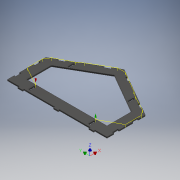
# Autodesk Inventor part: BA15
Saved by Autodesk Inventor 2017 (Build 210142000, 142)
## iProperties
Created: 2019-05-29
Part Number: BA15
Material: Wood (Cherry)
Document SubType Name: Modeling
Designer: Dell
Density: 0.63 g/cm^3
Appearance: Smooth - Black
Mass: 254.003 g
Surface Area: 1468.73 cm^2
Volume: 403.179 cm^3
Author: Dell
Autodesk Inventor part; units mm, degrees
ref_plane "YZ Plane" through (0, 0, 0) normal (1, 0, 0) x (0, 1, 0)
ref_plane "XZ Plane" through (0, 0, 0) normal (0, 1, 0) x (-1, 0, 0)
ref_plane "XY Plane" through (0, 0, 0) normal (0, 0, 1) x (1, 0, 0)
sketch "Sketch1" plane through (0, 0, 0) normal (0, 0, 1) x (1, 0, 0)
  line L0 (0, 0) -> (0, 201.9592)
  line L1 (0, 201.9592) -> (262.89, 353.7388)
  line L2 (262.89, 353.7388) -> (525.78, 201.9592)
  line L3 (525.78, 201.9592) -> (525.78, 0)
  line L4 (525.78, 0) -> (0, 0)
  point P0 (262.89, 0)
  dimension "d0" = 525.78
  dimension "d1" = 120
  dimension "d2" = 201.9592
  constraints: 10 end point, 1 horizontal alignment, 1 midpoint, 1 parallel, 1 perpendicular, 1 vertical, 1 vertical alignment
  measures "d0" distance of L3.end L0.start
  measures "d1" angle of L2 L1
  measures "d2" distance of L0.start L0.end
extrude "Extrusion1" add sketch "Sketch1" along normal blind 6.35
sketch "Sketch3" plane through (0, 0, 6.35) normal (0, 0, 1) x (1, 0, 0)
  line L0 (50.8, 180.4886) -> (474.98, 180.4886)
  line L1 (474.98, 180.4886) -> (474.98, 50.8)
  line L2 (474.98, 50.8) -> (50.8, 50.8)
  line L3 (50.8, 50.8) -> (50.8, 180.4886)
  line L4 (0, 201.9592) -> (0, 0) projected
  line L5 (50.8, 180.4886) -> (262.89, 302.9388)
  line L6 (262.89, 302.9388) -> (474.98, 180.4886)
  line L7 (525.78, 0) -> (0, 0) projected
  point P0 (262.89, 353.7388)
  point P1 (262.89, 180.4886)
  dimension "d15" = 120
  dimension "d16" = 50.8
  dimension "d17" = 50.8
  dimension "d18" = 50.8
  constraints: 12 end point, 2 parallel, 2 vertical alignment, 1 horizontal, 1 midpoint, 1 perpendicular
  measures "d15" angle of L6 L5
  measures "d16" distance between parallel lines of L4 L3
  measures "d17" distance between parallel lines of L7 L2
  measures "d18" distance of point (262.89, 353.739) L5.end
extrude "Extrusion3" cut sketch "Sketch3" against normal through all
sketch "Sketch4" plane through (0, 0, 6.35) normal (0, 0, 1) x (1, 0, 0)
  line L0 (525.78, 163.8592) -> (518.16, 163.8592)
  line L1 (518.16, 163.8592) -> (518.16, 138.4592)
  line L2 (518.16, 138.4592) -> (525.78, 138.4592)
  line L3 (525.78, 138.4592) -> (525.78, 163.8592)
  line L4 (525.78, 201.9592) -> (525.78, 0) projected
  line L5 (525.78, 36.8592) -> (518.16, 36.8592)
  line L6 (518.16, 36.8592) -> (518.16, 62.2592)
  line L7 (518.16, 62.2592) -> (525.78, 62.2592)
  line L8 (525.78, 62.2592) -> (525.78, 36.8592)
  line L9 (518.16, 151.1592) -> (518.16, 49.5592) construction
  line L10 (262.89, 353.7388) -> (262.89, 385.1225)
  line L11 (0, 163.8592) -> (7.62, 163.8592)
  line L12 (7.62, 163.8592) -> (7.62, 138.4592)
  line L13 (7.62, 138.4592) -> (0, 138.4592)
  line L14 (0, 138.4592) -> (0, 163.8592)
  line L15 (0, 201.9592) -> (0, 0)
  line L16 (0, 36.8592) -> (7.62, 36.8592)
  line L17 (7.62, 36.8592) -> (7.62, 62.2592)
  line L18 (7.62, 62.2592) -> (0, 62.2592)
  line L19 (0, 62.2592) -> (0, 36.8592)
  line L20 (7.62, 151.1592) -> (7.62, 49.5592) construction
  point P0 (0, 0)
  dimension "d19" = 38.1
  dimension "d20" = 25.4
  dimension "d21" = 25.4
  dimension "d22" = 7.62
  dimension "d23" = 101.6
  constraints: 40 end point, 12 symmetric about line, 4 parallel, 4 point on line, 2 horizontal, 2 midpoint, 2 perpendicular, 1 vertical, 1 vertical alignment
  measures "d19" vertical distance of L4.start L0.end
  measures "d20" distance of L0.end L1.end
  measures "d21" distance of L5.end L6.end
  measures "d22" distance of L0.start L0.end
  measures "d23" distance of L9.start L9.end
extrude "Extrusion4" cut sketch "Sketch4" against normal through all
sketch "Sketch5" plane through (0, 0, 6.35) normal (0, 0, 1) x (1, 0, 0)
  line L0 (302.5368, 322.0499) -> (306.3468, 328.649)
  line L1 (306.3468, 328.649) -> (328.3439, 315.949)
  line L2 (328.3439, 315.949) -> (324.5339, 309.3499)
  line L3 (324.5339, 309.3499) -> (302.5368, 322.0499)
  line L4 (460.3261, 239.749) -> (456.5161, 233.1499)
  line L5 (456.5161, 233.1499) -> (478.5132, 220.4499)
  line L6 (478.5132, 220.4499) -> (482.3232, 227.049)
  line L7 (482.3232, 227.049) -> (460.3261, 239.749)
  line L8 (525.78, 201.9592) -> (262.89, 353.7388) construction
  line L9 (313.5353, 315.6999) -> (467.5147, 226.7999) construction
  line L10 (390.525, 271.2499) -> (394.335, 277.849) construction
  line L11 (262.89, 353.7388) -> (525.78, 201.9592) construction
  line L12 (262.89, 353.7388) -> (262.89, 420.8284)
  line L13 (223.2432, 322.0499) -> (219.4332, 328.649)
  line L14 (219.4332, 328.649) -> (197.4361, 315.949)
  line L15 (197.4361, 315.949) -> (201.2461, 309.3499)
  line L16 (201.2461, 309.3499) -> (223.2432, 322.0499)
  line L17 (65.4539, 239.749) -> (69.2639, 233.1499)
  line L18 (69.2639, 233.1499) -> (47.2668, 220.4499)
  line L19 (47.2668, 220.4499) -> (43.4568, 227.049)
  line L20 (43.4568, 227.049) -> (65.4539, 239.749)
  line L21 (212.2447, 315.6999) -> (58.2653, 226.7999) construction
  line L22 (135.255, 271.2499) -> (131.445, 277.849) construction
  point P0 (0, 0)
  point P1 (0, 201.9592)
  dimension "d26" = 7.62
  dimension "d27" = 25.4
  dimension "d28" = 25.4
  dimension "d30" = 152.4
  constraints: 42 end point, 13 symmetric about line, 5 midpoint, 5 parallel, 4 perpendicular, 3 point on line, 1 vertical
  measures "d26" distance of L0.start L0.end
  measures "d27" distance of L2.end L0.start
  measures "d28" distance of L4.end L5.end
  measures "d30" distance of L4.end L2.end
extrude "Extrusion5" cut sketch "Sketch5" against normal through all
sketch "Sketch6" plane through (0, 0, 6.35) normal (0, 0, 1) x (1, 0, 0)
  line L0 (525.78, 0) -> (0, 0) projected
  line L1 (250.19, 0) -> (275.59, 0)
  line L2 (275.59, 0) -> (275.59, -7.62)
  line L3 (275.59, -7.62) -> (250.19, -7.62)
  line L4 (250.19, -7.62) -> (250.19, 0)
  line L5 (62.69, 0) -> (88.09, 0)
  line L6 (88.09, 0) -> (88.09, -7.62)
  line L7 (88.09, -7.62) -> (62.69, -7.62)
  line L8 (62.69, -7.62) -> (62.69, 0)
  line L9 (437.69, 0) -> (463.09, 0)
  line L10 (463.09, 0) -> (463.09, -7.62)
  line L11 (463.09, -7.62) -> (437.69, -7.62)
  line L12 (437.69, -7.62) -> (437.69, 0)
  line L13 (75.39, -7.62) -> (450.39, -7.62) construction
  point P0 (262.89, 0)
  point P1 (262.89, -7.62)
  dimension "d33" = 25.4
  dimension "d34" = 7.62
  dimension "d35" = 25.4
  dimension "d36" = 25.4
  dimension "d37" = 375
  constraints: 26 end point, 6 midpoint, 6 parallel, 3 horizontal, 3 perpendicular, 3 point on line, 2 horizontal alignment
  measures "d33" distance of L2.end L3.end
  measures "d34" distance of L1.end L2.end
  measures "d35" distance of L6.end L7.end
  measures "d36" distance of L10.end L11.end
  measures "d37" distance of L13.start L13.end
extrude "Extrusion6" add sketch "Sketch6" against normal blind 6.35
sketch "Sketch7" plane through (0, 0, 6.35) normal (0, 0, 1) x (1, 0, 0)
  line L0 (101.6, 245.2342) -> (107.95, 245.2342)
  line L1 (107.95, 245.2342) -> (107.95, 219.8342)
  line L2 (107.95, 219.8342) -> (101.6, 219.8342)
  line L3 (101.6, 219.8342) -> (101.6, 245.2342)
  line L4 (107.95, 38.1) -> (101.6, 38.1)
  line L5 (101.6, 38.1) -> (101.6, 12.7)
  line L6 (101.6, 12.7) -> (107.95, 12.7)
  line L7 (107.95, 12.7) -> (107.95, 38.1)
  line L8 (0, 0) -> (62.69, 0) projected
  line L9 (0, 36.8592) -> (0, 0) projected
  line L10 (262.89, 353.7388) -> (262.89, 392.9766)
  line L11 (424.18, 245.2342) -> (417.83, 245.2342)
  line L12 (417.83, 245.2342) -> (417.83, 219.8342)
  line L13 (417.83, 219.8342) -> (424.18, 219.8342)
  line L14 (424.18, 219.8342) -> (424.18, 245.2342)
  line L15 (417.83, 38.1) -> (424.18, 38.1)
  line L16 (424.18, 38.1) -> (424.18, 12.7)
  line L17 (424.18, 12.7) -> (417.83, 12.7)
  line L18 (417.83, 12.7) -> (417.83, 38.1)
  point P0 (104.775, 219.8342)
  point P1 (104.775, 38.1)
  point P2 (421.005, 219.8342)
  point P3 (421.005, 38.1)
  point P4 (463.09, 0)
  dimension "d40" = 6.35
  dimension "d41" = 25.4
  dimension "d42" = 12.7
  dimension "d43" = 25.4
  dimension "d44" = 101.6
  dimension "d45" = 181.7342
  constraints: 34 end point, 11 symmetric about line, 4 parallel, 4 point on line, 2 horizontal, 2 midpoint, 2 perpendicular, 2 vertical alignment, 1 vertical
  measures "d40" distance of L1.end L2.end
  measures "d41" distance of L0.end L1.end
  measures "d42" distance from line of L8 L5.end
  measures "d43" distance of L6.end L4.start
  measures "d44" distance between parallel lines of L9 L5
  measures "d45" distance of point (104.775, 38.1) point (104.775, 219.834)
extrude "Extrusion7" cut sketch "Sketch7" against normal through all
sketch "Sketch8" plane through (0, 0, 6.35) normal (0, 0, 1) x (1, 0, 0)
  circle A0 centre (3.175, 100.3592) radius 2.25
  line L0 (417.83, 219.8342) -> (417.83, 245.2342) construction
  line L1 (417.83, 245.2342) -> (424.18, 245.2342) construction
  line L2 (424.18, 245.2342) -> (424.18, 219.8342) construction
  line L3 (424.18, 219.8342) -> (417.83, 219.8342) construction
  line L4 (101.6, 219.8342) -> (101.6, 245.2342) construction
  line L5 (101.6, 245.2342) -> (107.95, 245.2342) construction
  line L6 (107.95, 245.2342) -> (107.95, 219.8342) construction
  line L7 (107.95, 219.8342) -> (101.6, 219.8342) construction
  line L8 (101.6, 12.7) -> (101.6, 38.1) construction
  line L9 (101.6, 38.1) -> (107.95, 38.1) construction
  line L10 (107.95, 38.1) -> (107.95, 12.7) construction
  line L11 (107.95, 12.7) -> (101.6, 12.7) construction
  line L12 (417.83, 12.7) -> (417.83, 38.1) construction
  line L13 (417.83, 38.1) -> (424.18, 38.1) construction
  line L14 (424.18, 38.1) -> (424.18, 12.7) construction
  line L15 (424.18, 12.7) -> (417.83, 12.7) construction
  line L16 (50.8, 50.8) -> (50.8, 180.4886) construction
  line L17 (50.8, 180.4886) -> (262.89, 302.9388) construction
  line L18 (262.89, 302.9388) -> (474.98, 180.4886) construction
  line L19 (474.98, 180.4886) -> (474.98, 50.8) construction
  line L20 (474.98, 50.8) -> (50.8, 50.8) construction
  line L21 (219.4332, 328.649) -> (223.2432, 322.0499) construction
  line L22 (223.2432, 322.0499) -> (201.2461, 309.3499) construction
  line L23 (201.2461, 309.3499) -> (197.4361, 315.949) construction
  line L24 (197.4361, 315.949) -> (65.4539, 239.749) construction
  line L25 (65.4539, 239.749) -> (69.2639, 233.1499) construction
  line L26 (69.2639, 233.1499) -> (47.2668, 220.4499) construction
  line L27 (47.2668, 220.4499) -> (43.4568, 227.049) construction
  line L28 (43.4568, 227.049) -> (0, 201.9592) construction
  line L29 (0, 201.9592) -> (0, 163.8592) construction
  line L30 (0, 163.8592) -> (7.62, 163.8592) construction
  line L31 (7.62, 163.8592) -> (7.62, 138.4592) construction
  line L32 (7.62, 138.4592) -> (0, 138.4592) construction
  line L33 (0, 138.4592) -> (0, 62.2592) construction
  line L34 (0, 62.2592) -> (7.62, 62.2592) construction
  line L35 (7.62, 62.2592) -> (7.62, 36.8592) construction
  line L36 (7.62, 36.8592) -> (0, 36.8592) construction
  line L37 (0, 36.8592) -> (0, 0) construction
  line L38 (0, 0) -> (62.69, 0) construction
  line L39 (62.69, 0) -> (62.69, -7.62) construction
  line L40 (62.69, -7.62) -> (88.09, -7.62) construction
  line L41 (88.09, -7.62) -> (88.09, 0) construction
  line L42 (88.09, 0) -> (250.19, 0) construction
  line L43 (250.19, 0) -> (250.19, -7.62) construction
  line L44 (250.19, -7.62) -> (275.59, -7.62) construction
  line L45 (275.59, -7.62) -> (275.59, 0) construction
  line L46 (275.59, 0) -> (437.69, 0) construction
  line L47 (437.69, 0) -> (437.69, -7.62) construction
  line L48 (437.69, -7.62) -> (463.09, -7.62) construction
  line L49 (463.09, -7.62) -> (463.09, 0) construction
  line L50 (463.09, 0) -> (525.78, 0) construction
  line L51 (525.78, 0) -> (525.78, 36.8592) construction
  line L52 (525.78, 36.8592) -> (518.16, 36.8592) construction
  line L53 (518.16, 36.8592) -> (518.16, 62.2592) construction
  line L54 (518.16, 62.2592) -> (525.78, 62.2592) construction
  line L55 (525.78, 62.2592) -> (525.78, 138.4592) construction
  line L56 (525.78, 138.4592) -> (518.16, 138.4592) construction
  line L57 (518.16, 138.4592) -> (518.16, 163.8592) construction
  line L58 (518.16, 163.8592) -> (525.78, 163.8592) construction
  line L59 (525.78, 163.8592) -> (525.78, 201.9592) construction
  line L60 (525.78, 201.9592) -> (482.3232, 227.049) construction
  line L61 (482.3232, 227.049) -> (478.5132, 220.4499) construction
  line L62 (478.5132, 220.4499) -> (456.5161, 233.1499) construction
  line L63 (456.5161, 233.1499) -> (460.3261, 239.749) construction
  line L64 (460.3261, 239.749) -> (328.3439, 315.949) construction
  line L65 (328.3439, 315.949) -> (324.5339, 309.3499) construction
  line L66 (324.5339, 309.3499) -> (302.5368, 322.0499) construction
  line L67 (302.5368, 322.0499) -> (306.3468, 328.649) construction
  line L68 (306.3468, 328.649) -> (262.89, 353.7388) construction
  line L69 (262.89, 353.7388) -> (219.4332, 328.649) construction
  line L70 (3.175, 65.4342) -> (3.175, 135.2842) construction
  line L71 (3.175, 135.2842) -> (10.795, 135.2842) construction
  line L72 (10.795, 135.2842) -> (10.795, 167.0342) construction
  line L73 (10.795, 167.0342) -> (3.175, 167.0342) construction
  line L74 (3.175, 167.0342) -> (3.175, 200.1261) construction
  line L75 (3.175, 200.1261) -> (42.2947, 222.7119) construction
  line L76 (42.2947, 222.7119) -> (46.1047, 216.1128) construction
  line L77 (46.1047, 216.1128) -> (73.601, 231.9878) construction
  line L78 (73.601, 231.9878) -> (69.791, 238.5869) construction
  line L79 (69.791, 238.5869) -> (196.274, 311.6119) construction
  line L80 (196.274, 311.6119) -> (200.084, 305.0128) construction
  line L81 (200.084, 305.0128) -> (227.5803, 320.8878) construction
  line L82 (227.5803, 320.8878) -> (223.7703, 327.4869) construction
  line L83 (223.7703, 327.4869) -> (262.89, 350.0727) construction
  line L84 (262.89, 350.0727) -> (302.0097, 327.4869) construction
  line L85 (302.0097, 327.4869) -> (298.1997, 320.8878) construction
  line L86 (298.1997, 320.8878) -> (325.696, 305.0128) construction
  line L87 (325.696, 305.0128) -> (329.506, 311.6119) construction
  line L88 (329.506, 311.6119) -> (455.989, 238.5869) construction
  line L89 (455.989, 238.5869) -> (452.179, 231.9878) construction
  line L90 (452.179, 231.9878) -> (479.6753, 216.1128) construction
  line L91 (479.6753, 216.1128) -> (483.4853, 222.7119) construction
  line L92 (483.4853, 222.7119) -> (522.605, 200.1261) construction
  line L93 (522.605, 200.1261) -> (522.605, 167.0342) construction
  line L94 (522.605, 167.0342) -> (514.985, 167.0342) construction
  line L95 (514.985, 167.0342) -> (514.985, 135.2842) construction
  line L96 (514.985, 135.2842) -> (522.605, 135.2842) construction
  line L97 (522.605, 135.2842) -> (522.605, 65.4342) construction
  line L98 (522.605, 65.4342) -> (514.985, 65.4342) construction
  line L99 (514.985, 65.4342) -> (514.985, 33.6842) construction
  line L100 (514.985, 33.6842) -> (522.605, 33.6842) construction
  line L101 (522.605, 33.6842) -> (522.605, 3.175) construction
  line L102 (522.605, 3.175) -> (459.915, 3.175) construction
  line L103 (459.915, 3.175) -> (459.915, -4.445) construction
  line L104 (459.915, -4.445) -> (440.865, -4.445) construction
  line L105 (440.865, -4.445) -> (440.865, 3.175) construction
  line L106 (440.865, 3.175) -> (272.415, 3.175) construction
  line L107 (272.415, 3.175) -> (272.415, -4.445) construction
  line L108 (272.415, -4.445) -> (253.365, -4.445) construction
  line L109 (253.365, -4.445) -> (253.365, 3.175) construction
  line L110 (253.365, 3.175) -> (84.915, 3.175) construction
  line L111 (84.915, 3.175) -> (84.915, -4.445) construction
  line L112 (84.915, -4.445) -> (65.865, -4.445) construction
  line L113 (65.865, -4.445) -> (65.865, 3.175) construction
  line L114 (65.865, 3.175) -> (3.175, 3.175) construction
  line L115 (3.175, 3.175) -> (3.175, 33.6842) construction
  line L116 (3.175, 33.6842) -> (10.795, 33.6842) construction
  line L117 (10.795, 33.6842) -> (10.795, 65.4342) construction
  line L118 (10.795, 65.4342) -> (3.175, 65.4342) construction
  circle A1 centre (3.175, 183.5802) radius 2.25
  circle A2 centre (22.7348, 211.419) radius 2.25
  circle A3 centre (133.0325, 275.0994) radius 2.25
  circle A4 centre (243.3302, 338.7798) radius 2.25
  circle A5 centre (282.4498, 338.7798) radius 2.25
  circle A6 centre (392.7475, 275.0994) radius 2.25
  circle A7 centre (503.0452, 211.419) radius 2.25
  circle A8 centre (522.605, 100.3592) radius 2.25
  circle A9 centre (522.605, 183.5802) radius 2.25
  circle A10 centre (421.005, 44.45) radius 2.25
  circle A11 centre (104.775, 44.45) radius 2.25
  circle A12 centre (104.775, 253.8426) radius 2.25
  circle A13 centre (421.005, 253.8426) radius 2.25
  line L119 (417.83, 245.2342) -> (424.18, 245.2342) construction
  line L120 (421.005, 245.2342) -> (421.005, 262.4511) construction
  line L121 (104.775, 245.2342) -> (104.775, 262.4511) construction
  line L122 (101.6, 38.1) -> (107.95, 38.1) construction
  line L123 (104.775, 38.1) -> (104.775, 50.8) construction
  line L124 (50.8, 50.8) -> (474.98, 50.8) construction
  line L125 (424.18, 38.1) -> (417.83, 38.1) construction
  line L126 (421.005, 38.1) -> (421.005, 50.8) construction
  point P0 (104.775, 44.45)
  dimension "d48" = 4.5
  dimension "d49" = 3.175
  dimension "d51" = 4.5
  dimension "d52" = 4.5
  dimension "d53" = 4.5
  dimension "d54" = 4.5
  dimension "d55" = 4.5
  dimension "d56" = 4.5
  dimension "d57" = 4.5
  dimension "d58" = 4.5
  dimension "d59" = 4.5
  dimension "d62" = 4.5
  dimension "d63" = 4.5
  dimension "d64" = 4.5
  dimension "d65" = 4.5
  constraints: 106 end point, 18 midpoint, 14 centre point, 6 point on line, 4 coincident, 1 parallel, 1 perpendicular, 48 other
  measures "d48" diameter of A0
  measures "d49" distance between parallel lines of L33 L70
  measures "d51" diameter of A1
  measures "d52" diameter of A2
  measures "d53" diameter of A3
  measures "d54" diameter of A4
  measures "d55" diameter of A5
  measures "d56" diameter of A6
  measures "d57" diameter of A7
  measures "d58" diameter of A8
  measures "d59" diameter of A9
  measures "d62" diameter of A10
  measures "d63" diameter of A11
  measures "d64" diameter of A12
  measures "d65" diameter of A13
extrude "Extrusion8" cut sketch "Sketch8" against normal through all
sketch "Sketch10" plane through (0, 0, 6.35) normal (0, 0, 1) x (1, 0, 0)
  circle A0 centre (104.775, 253.8426) radius 2.25 construction
  circle A1 centre (421.005, 44.45) radius 2.25 construction
  circle A2 centre (522.605, 100.3592) radius 2.25 construction
  circle A3 centre (392.7475, 275.0994) radius 2.25 construction
  circle A4 centre (243.3302, 338.7798) radius 2.25 construction
  circle A5 centre (22.7348, 211.419) radius 2.25 construction
  circle A6 centre (3.175, 100.3592) radius 2.25 construction
  circle A7 centre (3.175, 183.5802) radius 2.25 construction
  circle A8 centre (133.0325, 275.0994) radius 2.25 construction
  circle A9 centre (282.4498, 338.7798) radius 2.25 construction
  circle A10 centre (503.0452, 211.419) radius 2.25 construction
  circle A11 centre (522.605, 183.5802) radius 2.25 construction
  circle A12 centre (104.775, 44.45) radius 2.25 construction
  circle A13 centre (421.005, 253.8426) radius 2.25 construction
  line L0 (417.83, 219.8342) -> (417.83, 245.2342) construction
  line L1 (417.83, 245.2342) -> (424.18, 245.2342) construction
  line L2 (424.18, 245.2342) -> (424.18, 219.8342) construction
  line L3 (424.18, 219.8342) -> (417.83, 219.8342) construction
  line L4 (101.6, 219.8342) -> (101.6, 245.2342) construction
  line L5 (101.6, 245.2342) -> (107.95, 245.2342) construction
  line L6 (107.95, 245.2342) -> (107.95, 219.8342) construction
  line L7 (107.95, 219.8342) -> (101.6, 219.8342) construction
  line L8 (101.6, 12.7) -> (101.6, 38.1) construction
  line L9 (101.6, 38.1) -> (107.95, 38.1) construction
  line L10 (107.95, 38.1) -> (107.95, 12.7) construction
  line L11 (107.95, 12.7) -> (101.6, 12.7) construction
  line L12 (417.83, 12.7) -> (417.83, 38.1) construction
  line L13 (417.83, 38.1) -> (424.18, 38.1) construction
  line L14 (424.18, 38.1) -> (424.18, 12.7) construction
  line L15 (424.18, 12.7) -> (417.83, 12.7) construction
  line L16 (50.8, 50.8) -> (50.8, 180.4886) construction
  line L17 (50.8, 180.4886) -> (262.89, 302.9388) construction
  line L18 (262.89, 302.9388) -> (474.98, 180.4886) construction
  line L19 (474.98, 180.4886) -> (474.98, 50.8) construction
  line L20 (474.98, 50.8) -> (50.8, 50.8) construction
  line L21 (219.4332, 328.649) -> (223.2432, 322.0499) construction
  line L22 (223.2432, 322.0499) -> (201.2461, 309.3499) construction
  line L23 (201.2461, 309.3499) -> (197.4361, 315.949) construction
  line L24 (197.4361, 315.949) -> (65.4539, 239.749) construction
  line L25 (65.4539, 239.749) -> (69.2639, 233.1499) construction
  line L26 (69.2639, 233.1499) -> (47.2668, 220.4499) construction
  line L27 (47.2668, 220.4499) -> (43.4568, 227.049) construction
  line L28 (43.4568, 227.049) -> (0, 201.9592) construction
  line L29 (0, 201.9592) -> (0, 163.8592) construction
  line L30 (0, 163.8592) -> (7.62, 163.8592) construction
  line L31 (7.62, 163.8592) -> (7.62, 138.4592) construction
  line L32 (7.62, 138.4592) -> (0, 138.4592) construction
  line L33 (0, 138.4592) -> (0, 62.2592) construction
  line L34 (0, 62.2592) -> (7.62, 62.2592) construction
  line L35 (7.62, 62.2592) -> (7.62, 36.8592) construction
  line L36 (7.62, 36.8592) -> (0, 36.8592) construction
  line L37 (0, 36.8592) -> (0, 0) construction
  line L38 (0, 0) -> (62.69, 0) construction
  line L39 (62.69, 0) -> (62.69, -7.62) construction
  line L40 (62.69, -7.62) -> (88.09, -7.62) construction
  line L41 (88.09, -7.62) -> (88.09, 0) construction
  line L42 (88.09, 0) -> (250.19, 0) construction
  line L43 (250.19, 0) -> (250.19, -7.62) construction
  line L44 (250.19, -7.62) -> (275.59, -7.62) construction
  line L45 (275.59, -7.62) -> (275.59, 0) construction
  line L46 (275.59, 0) -> (437.69, 0) construction
  line L47 (437.69, 0) -> (437.69, -7.62) construction
  line L48 (437.69, -7.62) -> (463.09, -7.62) construction
  line L49 (463.09, -7.62) -> (463.09, 0) construction
  line L50 (463.09, 0) -> (525.78, 0) construction
  line L51 (525.78, 0) -> (525.78, 36.8592) construction
  line L52 (525.78, 36.8592) -> (518.16, 36.8592) construction
  line L53 (518.16, 36.8592) -> (518.16, 62.2592) construction
  line L54 (518.16, 62.2592) -> (525.78, 62.2592) construction
  line L55 (525.78, 62.2592) -> (525.78, 138.4592) construction
  line L56 (525.78, 138.4592) -> (518.16, 138.4592) construction
  line L57 (518.16, 138.4592) -> (518.16, 163.8592) construction
  line L58 (518.16, 163.8592) -> (525.78, 163.8592) construction
  line L59 (525.78, 163.8592) -> (525.78, 201.9592) construction
  line L60 (525.78, 201.9592) -> (482.3232, 227.049) construction
  line L61 (482.3232, 227.049) -> (478.5132, 220.4499) construction
  line L62 (478.5132, 220.4499) -> (456.5161, 233.1499) construction
  line L63 (456.5161, 233.1499) -> (460.3261, 239.749) construction
  line L64 (460.3261, 239.749) -> (328.3439, 315.949) construction
  line L65 (328.3439, 315.949) -> (324.5339, 309.3499) construction
  line L66 (324.5339, 309.3499) -> (302.5368, 322.0499) construction
  line L67 (302.5368, 322.0499) -> (306.3468, 328.649) construction
  line L68 (306.3468, 328.649) -> (262.89, 353.7388) construction
  line L69 (262.89, 353.7388) -> (219.4332, 328.649) construction
  line L70 (0, 138.4592) -> (0, 62.2592) projected
  line L71 (0, 63.5292) -> (7.62, 63.5292)
  line L72 (7.62, 63.5292) -> (7.62, 35.5892)
  line L73 (7.62, 35.5892) -> (0, 35.5892)
  line L74 (0, 35.5892) -> (0, 63.5292)
  line L75 (0, 137.1892) -> (7.62, 137.1892)
  line L76 (7.62, 137.1892) -> (7.62, 165.1292)
  line L77 (7.62, 165.1292) -> (0, 165.1292)
  line L78 (0, 165.1292) -> (0, 137.1892)
  line L79 (100.33, 39.37) -> (109.22, 39.37)
  line L80 (109.22, 39.37) -> (109.22, 11.43)
  line L81 (109.22, 11.43) -> (100.33, 11.43)
  line L82 (100.33, 11.43) -> (100.33, 39.37)
  line L83 (416.56, 39.37) -> (425.45, 39.37)
  line L84 (425.45, 39.37) -> (425.45, 11.43)
  line L85 (425.45, 11.43) -> (416.56, 11.43)
  line L86 (416.56, 11.43) -> (416.56, 39.37)
  line L87 (525.78, 36.8592) -> (525.78, 0) projected
  line L88 (525.78, 35.5892) -> (518.16, 35.5892)
  line L89 (518.16, 35.5892) -> (518.16, 63.5292)
  line L90 (518.16, 63.5292) -> (525.78, 63.5292)
  line L91 (525.78, 63.5292) -> (525.78, 35.5892)
  line L92 (525.78, 138.4592) -> (525.78, 62.2592) projected
  line L93 (525.78, 137.1892) -> (518.16, 137.1892)
  line L94 (518.16, 137.1892) -> (518.16, 165.1292)
  line L95 (518.16, 165.1292) -> (525.78, 165.1292)
  line L96 (525.78, 165.1292) -> (525.78, 137.1892)
  line L97 (100.33, 246.5042) -> (109.22, 246.5042)
  line L98 (109.22, 246.5042) -> (109.22, 218.5642)
  line L99 (109.22, 218.5642) -> (100.33, 218.5642)
  line L100 (100.33, 218.5642) -> (100.33, 246.5042)
  line L101 (416.56, 246.5042) -> (425.45, 246.5042)
  line L102 (425.45, 246.5042) -> (425.45, 218.5642)
  line L103 (425.45, 218.5642) -> (416.56, 218.5642)
  line L104 (416.56, 218.5642) -> (416.56, 246.5042)
  line L105 (43.4568, 227.049) -> (0, 201.9592) projected
  line L106 (65.4539, 239.749) -> (197.4361, 315.949) projected
  line L107 (42.357, 226.414) -> (66.5537, 240.384)
  line L108 (66.5537, 240.384) -> (70.3637, 233.7849)
  line L109 (70.3637, 233.7849) -> (46.167, 219.8149)
  line L110 (46.167, 219.8149) -> (42.357, 226.414)
  line L111 (219.4332, 328.649) -> (262.89, 353.7388) projected
  line L112 (196.3363, 315.314) -> (220.533, 329.284)
  line L113 (220.533, 329.284) -> (224.343, 322.6849)
  line L114 (224.343, 322.6849) -> (200.1463, 308.7149)
  line L115 (200.1463, 308.7149) -> (196.3363, 315.314)
  line L116 (262.89, 302.9388) -> (262.89, 353.7388)
  line L117 (306.3468, 328.649) -> (302.5368, 322.0499) construction
  line L118 (302.5368, 322.0499) -> (324.5339, 309.3499) construction
  line L119 (324.5339, 309.3499) -> (328.3439, 315.949) construction
  line L120 (460.3261, 239.749) -> (456.5161, 233.1499) construction
  line L121 (456.5161, 233.1499) -> (478.5132, 220.4499) construction
  line L122 (478.5132, 220.4499) -> (482.3232, 227.049) construction
  line L123 (483.423, 226.414) -> (459.2263, 240.384)
  line L124 (459.2263, 240.384) -> (455.4163, 233.7849)
  line L125 (455.4163, 233.7849) -> (479.613, 219.8149)
  line L126 (479.613, 219.8149) -> (483.423, 226.414)
  line L127 (329.4437, 315.314) -> (305.247, 329.284)
  line L128 (305.247, 329.284) -> (301.437, 322.6849)
  line L129 (301.437, 322.6849) -> (325.6337, 308.7149)
  line L130 (325.6337, 308.7149) -> (329.4437, 315.314)
  point P0 (107.95, 232.5342)
  point P1 (109.22, 232.5342)
  point P2 (104.775, 245.2342)
  point P3 (104.775, 246.5042)
  point P4 (421.005, 245.2342)
  point P5 (421.005, 246.5042)
  point P6 (417.83, 232.5342)
  point P7 (416.56, 232.5342)
  point P8 (518.16, 151.1592)
  point P9 (518.16, 151.1592)
  point P10 (518.16, 49.5592)
  point P11 (518.16, 49.5592)
  point P12 (421.005, 38.1)
  point P13 (421.005, 39.37)
  point P14 (104.775, 38.1)
  point P15 (104.775, 39.37)
  point P16 (416.56, 25.4)
  point P17 (417.83, 25.4)
  point P18 (101.6, 25.4)
  point P19 (100.33, 25.4)
  point P20 (7.62, 49.5592)
  point P21 (7.62, 49.5592)
  point P22 (7.62, 151.1592)
  point P23 (7.62, 151.1592)
  point P24 (212.2447, 315.6999)
  point P25 (58.2653, 226.7999)
  point P26 (313.5353, 315.6999)
  point P27 (467.5147, 226.7999)
  dimension "d66" = 1.27
  dimension "d67" = 1.27
  dimension "d68" = 1.27
  dimension "d69" = 1.27
  dimension "d70" = 1.27
  dimension "d71" = 1.27
  dimension "d72" = 1.27
  dimension "d73" = 1.27
  dimension "d74" = 1.27
  dimension "d75" = 1.27
  constraints: 110 end point, 28 midpoint, 20 parallel, 17 point on line, 10 perpendicular, 10 symmetric about line, 8 horizontal, 6 vertical alignment, 4 coincident, 4 horizontal alignment, 1 vertical
  measures "d66" distance between parallel lines of L77 L30
  measures "d67" distance between parallel lines of L71 L34
  measures "d68" distance between parallel lines of L79 L9
  measures "d69" distance between parallel lines of L80 L10
  measures "d70" distance between parallel lines of L84 L14
  measures "d71" distance between parallel lines of L102 L2
  measures "d72" distance between parallel lines of L101 L1
  measures "d73" distance between parallel lines of L98 L6
  measures "d74" distance between parallel lines of L108 L25
  measures "d75" distance between parallel lines of L115 L23
extrude "Extrusion9" cut sketch "Sketch10" against normal through all
sketch "Sketch12" plane through (0, 0, 6.35) normal (0, 0, 1) x (1, 0, 0)
  line L0 (50.8, 50.8) -> (50.8, 180.4886) construction
  line L1 (50.8, 180.4886) -> (262.89, 302.9388) construction
  line L2 (262.89, 302.9388) -> (474.98, 180.4886) construction
  line L3 (474.98, 180.4886) -> (474.98, 50.8) construction
  line L4 (474.98, 50.8) -> (50.8, 50.8) construction
  circle A0 centre (421.005, 253.8426) radius 2.25 construction
  circle A1 centre (104.775, 44.45) radius 2.25 construction
  circle A2 centre (522.605, 183.5802) radius 2.25 construction
  circle A3 centre (503.0452, 211.419) radius 2.25 construction
  circle A4 centre (282.4498, 338.7798) radius 2.25 construction
  circle A5 centre (133.0325, 275.0994) radius 2.25 construction
  circle A6 centre (3.175, 183.5802) radius 2.25 construction
  circle A7 centre (3.175, 100.3592) radius 2.25 construction
  circle A8 centre (22.7348, 211.419) radius 2.25 construction
  circle A9 centre (243.3302, 338.7798) radius 2.25 construction
  circle A10 centre (392.7475, 275.0994) radius 2.25 construction
  circle A11 centre (522.605, 100.3592) radius 2.25 construction
  circle A12 centre (421.005, 44.45) radius 2.25 construction
  circle A13 centre (104.775, 253.8426) radius 2.25 construction
  line L5 (416.56, 218.5642) -> (416.56, 246.5042) construction
  line L6 (416.56, 246.5042) -> (425.45, 246.5042) construction
  line L7 (425.45, 246.5042) -> (425.45, 218.5642) construction
  line L8 (425.45, 218.5642) -> (416.56, 218.5642) construction
  line L9 (416.56, 11.43) -> (416.56, 39.37) construction
  line L10 (416.56, 39.37) -> (425.45, 39.37) construction
  line L11 (425.45, 39.37) -> (425.45, 11.43) construction
  line L12 (425.45, 11.43) -> (416.56, 11.43) construction
  line L13 (100.33, 11.43) -> (100.33, 39.37) construction
  line L14 (100.33, 39.37) -> (109.22, 39.37) construction
  line L15 (109.22, 39.37) -> (109.22, 11.43) construction
  line L16 (109.22, 11.43) -> (100.33, 11.43) construction
  line L17 (100.33, 218.5642) -> (100.33, 246.5042) construction
  line L18 (100.33, 246.5042) -> (109.22, 246.5042) construction
  line L19 (109.22, 246.5042) -> (109.22, 218.5642) construction
  line L20 (109.22, 218.5642) -> (100.33, 218.5642) construction
  line L21 (483.423, 226.414) -> (479.613, 219.8149) construction
  line L22 (479.613, 219.8149) -> (455.4163, 233.7849) construction
  line L23 (455.4163, 233.7849) -> (459.2263, 240.384) construction
  line L24 (459.2263, 240.384) -> (329.4437, 315.314) construction
  line L25 (329.4437, 315.314) -> (325.6337, 308.7149) construction
  line L26 (325.6337, 308.7149) -> (301.437, 322.6849) construction
  line L27 (301.437, 322.6849) -> (305.247, 329.284) construction
  line L28 (305.247, 329.284) -> (262.89, 353.7388) construction
  line L29 (262.89, 353.7388) -> (220.533, 329.284) construction
  line L30 (220.533, 329.284) -> (224.343, 322.6849) construction
  line L31 (224.343, 322.6849) -> (200.1463, 308.7149) construction
  line L32 (200.1463, 308.7149) -> (196.3363, 315.314) construction
  line L33 (196.3363, 315.314) -> (66.5537, 240.384) construction
  line L34 (66.5537, 240.384) -> (70.3637, 233.7849) construction
  line L35 (70.3637, 233.7849) -> (46.167, 219.8149) construction
  line L36 (46.167, 219.8149) -> (42.357, 226.414) construction
  line L37 (42.357, 226.414) -> (0, 201.9592) construction
  line L38 (0, 201.9592) -> (0, 165.1292) construction
  line L39 (0, 165.1292) -> (7.62, 165.1292) construction
  line L40 (7.62, 165.1292) -> (7.62, 137.1892) construction
  line L41 (7.62, 137.1892) -> (0, 137.1892) construction
  line L42 (0, 137.1892) -> (0, 63.5292) construction
  line L43 (0, 63.5292) -> (7.62, 63.5292) construction
  line L44 (7.62, 63.5292) -> (7.62, 35.5892) construction
  line L45 (7.62, 35.5892) -> (0, 35.5892) construction
  line L46 (0, 35.5892) -> (0, 0) construction
  line L47 (0, 0) -> (62.69, 0) construction
  line L48 (62.69, 0) -> (62.69, -7.62) construction
  line L49 (62.69, -7.62) -> (88.09, -7.62) construction
  line L50 (88.09, -7.62) -> (88.09, 0) construction
  line L51 (88.09, 0) -> (250.19, 0) construction
  line L52 (250.19, 0) -> (250.19, -7.62) construction
  line L53 (250.19, -7.62) -> (275.59, -7.62) construction
  line L54 (275.59, -7.62) -> (275.59, 0) construction
  line L55 (275.59, 0) -> (437.69, 0) construction
  line L56 (437.69, 0) -> (437.69, -7.62) construction
  line L57 (437.69, -7.62) -> (463.09, -7.62) construction
  line L58 (463.09, -7.62) -> (463.09, 0) construction
  line L59 (463.09, 0) -> (525.78, 0) construction
  line L60 (525.78, 0) -> (525.78, 35.5892) construction
  line L61 (525.78, 35.5892) -> (518.16, 35.5892) construction
  line L62 (518.16, 35.5892) -> (518.16, 63.5292) construction
  line L63 (518.16, 63.5292) -> (525.78, 63.5292) construction
  line L64 (525.78, 63.5292) -> (525.78, 137.1892) construction
  line L65 (525.78, 137.1892) -> (518.16, 137.1892) construction
  line L66 (518.16, 137.1892) -> (518.16, 165.1292) construction
  line L67 (518.16, 165.1292) -> (525.78, 165.1292) construction
  line L68 (525.78, 165.1292) -> (525.78, 201.9592) construction
  line L69 (525.78, 201.9592) -> (483.423, 226.414) construction
  line L70 (63.4869, 241.2058) -> (197.158, 318.3808) construction
  line L71 (197.158, 318.3808) -> (200.968, 311.7817) construction
  line L72 (200.968, 311.7817) -> (221.2762, 323.5067) construction
  line L73 (221.2762, 323.5067) -> (217.4662, 330.1058) construction
  line L74 (217.4662, 330.1058) -> (262.89, 356.3312) construction
  line L75 (262.89, 356.3312) -> (308.3138, 330.1058) construction
  line L76 (308.3138, 330.1058) -> (304.5038, 323.5067) construction
  line L77 (304.5038, 323.5067) -> (324.812, 311.7817) construction
  line L78 (324.812, 311.7817) -> (328.622, 318.3808) construction
  line L79 (328.622, 318.3808) -> (462.2931, 241.2058) construction
  line L80 (462.2931, 241.2058) -> (458.4831, 234.6067) construction
  line L81 (458.4831, 234.6067) -> (478.7913, 222.8817) construction
  line L82 (478.7913, 222.8817) -> (482.6013, 229.4808) construction
  line L83 (482.6013, 229.4808) -> (528.0251, 203.2554) construction
  line L84 (528.0251, 203.2554) -> (528.0251, 162.8842) construction
  line L85 (528.0251, 162.8842) -> (520.4051, 162.8842) construction
  line L86 (520.4051, 162.8842) -> (520.4051, 139.4343) construction
  line L87 (520.4051, 139.4343) -> (528.0251, 139.4343) construction
  line L88 (528.0251, 139.4343) -> (528.0251, 61.2842) construction
  line L89 (528.0251, 61.2842) -> (520.4051, 61.2842) construction
  line L90 (520.4051, 61.2842) -> (520.4051, 37.8343) construction
  line L91 (520.4051, 37.8343) -> (528.0251, 37.8343) construction
  line L92 (528.0251, 37.8343) -> (528.0251, -2.2451) construction
  line L93 (528.0251, -2.2451) -> (465.3351, -2.2451) construction
  line L94 (465.3351, -2.2451) -> (465.3351, -9.8651) construction
  line L95 (465.3351, -9.8651) -> (435.4449, -9.8651) construction
  line L96 (435.4449, -9.8651) -> (435.4449, -2.2451) construction
  line L97 (435.4449, -2.2451) -> (277.8351, -2.2451) construction
  line L98 (277.8351, -2.2451) -> (277.8351, -9.8651) construction
  line L99 (277.8351, -9.8651) -> (247.9449, -9.8651) construction
  line L100 (247.9449, -9.8651) -> (247.9449, -2.2451) construction
  line L101 (247.9449, -2.2451) -> (90.3351, -2.2451) construction
  line L102 (90.3351, -2.2451) -> (90.3351, -9.8651) construction
  line L103 (90.3351, -9.8651) -> (60.4449, -9.8651) construction
  line L104 (60.4449, -9.8651) -> (60.4449, -2.2451) construction
  line L105 (60.4449, -2.2451) -> (-2.2451, -2.2451) construction
  line L106 (-2.2451, -2.2451) -> (-2.2451, 37.8343) construction
  line L107 (-2.2451, 37.8343) -> (5.3749, 37.8343) construction
  line L108 (5.3749, 37.8343) -> (5.3749, 61.2842) construction
  line L109 (5.3749, 61.2842) -> (-2.2451, 61.2842) construction
  line L110 (-2.2451, 61.2842) -> (-2.2451, 139.4343) construction
  line L111 (-2.2451, 139.4343) -> (5.3749, 139.4343) construction
  line L112 (5.3749, 139.4343) -> (5.3749, 162.8842) construction
  line L113 (5.3749, 162.8842) -> (-2.2451, 162.8842) construction
  line L114 (-2.2451, 162.8842) -> (-2.2451, 203.2554) construction
  line L115 (-2.2451, 203.2554) -> (43.1787, 229.4808) construction
  line L116 (43.1787, 229.4808) -> (46.9887, 222.8817) construction
  line L117 (46.9887, 222.8817) -> (67.2969, 234.6067) construction
  line L118 (67.2969, 234.6067) -> (63.4869, 241.2058) construction
  circle A14 centre (200.968, 311.7817) radius 3.175
  line L119 (200.1463, 308.7149) -> (224.343, 322.6849) projected
  circle A15 centre (221.2762, 323.5067) radius 3.175
  line L120 (301.437, 322.6849) -> (325.6337, 308.7149) projected
  circle A16 centre (304.5038, 323.5067) radius 3.175
  circle A17 centre (324.812, 311.7817) radius 3.175
  circle A18 centre (458.4831, 234.6067) radius 3.175
  line L121 (483.423, 226.414) -> (479.613, 219.8149) projected
  circle A19 centre (478.7913, 222.8817) radius 3.175
  line L122 (518.16, 165.1292) -> (518.16, 137.1892) projected
  circle A20 centre (520.4051, 162.8842) radius 3.175
  circle A21 centre (520.4051, 139.4343) radius 3.175
  line L123 (518.16, 63.5292) -> (518.16, 35.5892) projected
  circle A22 centre (520.4051, 61.2842) radius 3.175
  circle A23 centre (520.4051, 37.8343) radius 3.175
  circle A24 centre (465.3351, -2.2451) radius 3.175
  circle A25 centre (435.4449, -2.2451) radius 3.175
  circle A26 centre (277.8351, -2.2451) radius 3.175
  line L124 (250.19, 0) -> (88.09, 0) projected
  circle A27 centre (247.9449, -2.2451) radius 3.175
  circle A28 centre (90.3351, -2.2451) radius 3.175
  line L125 (62.69, -7.62) -> (62.69, 0) projected
  circle A29 centre (60.4449, -2.2451) radius 3.175
  circle A30 centre (5.3749, 37.8343) radius 3.175
  circle A31 centre (5.3749, 61.2842) radius 3.175
  line L126 (7.62, 137.1892) -> (7.62, 165.1292) projected
  circle A32 centre (5.3749, 139.4343) radius 3.175
  circle A33 centre (5.3749, 162.8842) radius 3.175
  circle A34 centre (46.9887, 222.8817) radius 3.175
  line L127 (46.167, 219.8149) -> (70.3637, 233.7849) projected
  circle A35 centre (67.2969, 234.6067) radius 3.175
  line L128 (102.5751, 244.2591) -> (102.5751, 220.8093) construction
  line L129 (102.5751, 220.8093) -> (106.9749, 220.8093) construction
  line L130 (106.9749, 220.8093) -> (106.9749, 244.2591) construction
  line L131 (106.9749, 244.2591) -> (102.5751, 244.2591) construction
  line L132 (102.5751, 37.1249) -> (102.5751, 13.6751) construction
  line L133 (102.5751, 13.6751) -> (106.9749, 13.6751) construction
  line L134 (106.9749, 13.6751) -> (106.9749, 37.1249) construction
  line L135 (106.9749, 37.1249) -> (102.5751, 37.1249) construction
  line L136 (418.8051, 37.1249) -> (418.8051, 13.6751) construction
  line L137 (418.8051, 13.6751) -> (423.2049, 13.6751) construction
  line L138 (423.2049, 13.6751) -> (423.2049, 37.1249) construction
  line L139 (423.2049, 37.1249) -> (418.8051, 37.1249) construction
  line L140 (418.8051, 244.2591) -> (418.8051, 220.8093) construction
  line L141 (418.8051, 220.8093) -> (423.2049, 220.8093) construction
  line L142 (423.2049, 220.8093) -> (423.2049, 244.2591) construction
  line L143 (423.2049, 244.2591) -> (418.8051, 244.2591) construction
  circle A36 centre (102.5751, 244.2591) radius 3.175
  circle A37 centre (106.9749, 244.2591) radius 3.175
  circle A38 centre (106.9749, 220.8093) radius 3.175
  line L144 (100.33, 218.5642) -> (109.22, 218.5642) projected
  circle A39 centre (102.5751, 220.8093) radius 3.175
  line L145 (100.33, 11.43) -> (100.33, 39.37) projected
  circle A40 centre (102.5751, 37.1249) radius 3.175
  line L146 (109.22, 39.37) -> (100.33, 39.37) projected
  circle A41 centre (106.9749, 37.1249) radius 3.175
  line L147 (109.22, 11.43) -> (100.33, 11.43) projected
  circle A42 centre (102.5751, 13.6751) radius 3.175
  circle A43 centre (106.9749, 13.6751) radius 3.175
  circle A44 centre (418.8051, 37.1249) radius 3.175
  circle A45 centre (423.2049, 37.1249) radius 3.175
  circle A46 centre (423.2049, 13.6751) radius 3.175
  line L148 (425.45, 11.43) -> (416.56, 11.43) projected
  circle A47 centre (418.8051, 13.6751) radius 3.175
  line L149 (425.45, 246.5042) -> (416.56, 246.5042) projected
  circle A48 centre (418.8051, 244.2591) radius 3.175
  circle A49 centre (423.2049, 244.2591) radius 3.175
  line L150 (416.56, 218.5642) -> (425.45, 218.5642) projected
  circle A50 centre (423.2049, 220.8093) radius 3.175
  circle A51 centre (418.8051, 220.8093) radius 3.175
  dimension "d78" = 6.35
  dimension "d79" = 6.35
  dimension "d80" = 6.35
  dimension "d81" = 6.35
  dimension "d82" = 6.35
  constraints: 131 end point, 36 coincident, 174 other
extrude "Extrusion10" cut sketch "Sketch12" along normal through all both and the other way through all
equation "\"d3\" = Panel_Thickness"
equation "\"d22\" = Panel_Thickness + Fit_Tolerance"
equation "\"d26\" = Panel_Thickness + Fit_Tolerance"
equation "\"d34\" = Panel_Thickness + Fit_Tolerance"
equation "\"d38\" = Panel_Thickness"
equation "\"d40\" = Panel_Thickness"
equation "\"d46\" = Panel_Thickness"
equation "\"d49\" = 0.5 * Panel_Thickness"
equation "\"d60\" = Panel_Thickness"
equation "\"d66\" = Fit_Tolerance"
equation "\"d67\" = Fit_Tolerance"
equation "\"d68\" = Fit_Tolerance"
equation "\"d69\" = Fit_Tolerance"
equation "\"d70\" = Fit_Tolerance"
equation "\"d71\" = Fit_Tolerance"
equation "\"d72\" = Fit_Tolerance"
equation "\"d73\" = Fit_Tolerance"
equation "\"d74\" = Fit_Tolerance"
equation "\"d75\" = Fit_Tolerance"
equation "\"d76\" = Panel_Thickness"
equation "\"d78\" = Tool_Dia"
equation "\"d79\" = d78"
equation "\"d80\" = d78"
equation "\"d81\" = d78"
equation "\"d82\" = d78"
equation "\"Panel_Thickness\" = 6.35"
equation "\"Fit_Tolerance\" = 1.27"
equation "\"Tool_Dia\" = 6.35"
body "Solid1"
